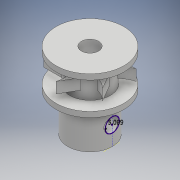
# Autodesk Inventor part: wheelSpindle
Saved by Autodesk Inventor 2018 (Build 220112000, 112)
## iProperties
Created: 2017-10-22
Part Number: wheelSpindle
Material: Generic
Document SubType Name: Modeling
Designer: Prakash
Density: 1 g/cm^3
Appearance: Default
Author: Prakash
Autodesk Inventor part; units mm, degrees
ref_plane "XZ Plane" through (0, 0, 0) normal (0, 1, 0) x (-1, 0, 0)
ref_plane "XY Plane" through (0, 0, 0) normal (0, 0, 1) x (1, 0, 0)
sketch "Sketch1" plane through (0, 0, 0) normal (0, 0, 1) x (1, 0, 0)
  circle A0 centre (0, 0) radius 7.5
  circle A1 centre (0, 0) radius 12.5
  circle A2 centre (0, 0) radius 3.175
  circle A3 centre (0, 0) radius 8.175
  dimension "d18" = 6.35
  dimension "d19" = 16.35
  dimension "d40" = 15
  dimension "d41" = 5
  constraints: 4 centre point, 4 coincident
  measures "d18" diameter of A2
  measures "d19" diameter of A3
  measures "d40" diameter of A0
  measures "d41" radial gap between concentric circles of A1 A0
extrude "Extrusion1" add sketch "Sketch1" along normal blind 14 contours A0 | A2
extrude "Extrusion2" add sketch "Sketch1" along normal blind 2 contours A1 | A3
sketch "Sketch2" plane through (0, 0, 14) normal (0, 0, 1) x (1, 0, 0)
  circle A0 centre (0, 0) radius 7.5 projected
  circle A1 centre (0, 0) radius 12.5 projected
extrude "Extrusion3" add sketch "Sketch2" against normal blind 2
ref_plane "Work Plane1" through (0, 0, 7) normal (0, 0, -1) x (-1, 0, 0)
extrude "Extrusion5" cut sketch "Sketch1" along normal up to surface (14 mm away) contours A2
extrude "Extrusion6" add sketch "Sketch1" against normal blind 14 contours A0 | A3
ref_plane "Work Plane2" through (8.175, 0, 0) normal (1, 0, 0) x (0, 1, 0)
sketch "Sketch9" plane through (0, 0, 7) normal (0, 0, -1) x (-1, 0, 0)
  circle A0 centre (0, 0) radius 7.5 projected
  line L0 (0, -7.5) -> (0, -12.5) construction
  circle A1 centre (0, 0) radius 12.5 projected
  arc A2 (0, -7.5) -> (0, -12.5) centre (7.5993, -10) ccw
  line L1 (0, -12.5) -> (-3.3398, -6.7154)
  circle A3 centre (0, 0) radius 7.5
  line L2 (6.4952, -3.75) -> (10.8253, -6.25) construction
  line L3 (10.8253, -6.25) -> (4.1458, -6.25)
  arc A4 (6.4952, -3.75) -> (10.8253, -6.25) centre (12.4599, 1.5812) ccw
  line L4 (6.4952, 3.75) -> (10.8253, 6.25) construction
  line L5 (10.8253, 6.25) -> (7.4855, 0.4654)
  arc A5 (6.4952, 3.75) -> (10.8253, 6.25) centre (4.8606, 11.5812) ccw
  line L6 (0, 7.5) -> (0, 12.5) construction
  line L7 (0, 12.5) -> (3.3398, 6.7154)
  arc A6 (0, 7.5) -> (0, 12.5) centre (-7.5993, 10) ccw
  line L8 (-6.4952, 3.75) -> (-10.8253, 6.25) construction
  line L9 (-10.8253, 6.25) -> (-4.1458, 6.25)
  arc A7 (-6.4952, 3.75) -> (-10.8253, 6.25) centre (-12.4599, -1.5812) ccw
  line L10 (-6.4952, -3.75) -> (-10.8253, -6.25) construction
  line L11 (-10.8253, -6.25) -> (-7.4855, -0.4654)
  arc A8 (-6.4952, -3.75) -> (-10.8253, -6.25) centre (-4.8606, -11.5812) ccw
  point P0 (0, -10)
  point P1 (8.6603, -5)
  point P2 (8.6603, 5)
  point P3 (0, 10)
  point P4 (-8.6603, 5)
  point P5 (-8.6603, -5)
  dimension "d58" = 8
  dimension "d59" = 30
  dimension "d62" = 360
  constraints: 24 end point, 12 point on circle, 7 centre point, 2 vertical, 1 coincident, 1 midpoint, 1 vertical alignment, 64 other
  measures "d58" radius of A2
  measures "d59" angle of L1 L0
extrude "Extrusion9" add sketch "Sketch9" along normal mid plane 4 contours A0 A5 L5 | A4 L3 A0 | A0 A6 L7 | A2 L1 A0 | L9 A0 A7 | L11 A0 A8
sketch "Sketch10" plane through (8.175, 0, 0) normal (1, 0, 0) x (0, 1, 0)
  line L0 (0, 0) -> (0, -14) construction
  line L1 (3.175, -14) -> (-3.175, -14) construction
  circle A0 centre (0, -7) radius 2.6543
  circle A1 centre (0, -7) radius 2.5273
  dimension "d67" = 5.3086
  dimension "d68" = 5.0546
  constraints: 2 centre point, 2 end point, 2 midpoint, 1 coincident
  measures "d67" diameter of A0
  measures "d68" diameter of A1
extrude "Extrusion10" cut sketch "Sketch10" against normal blind 3.81 contours A1
loft "Loft1" cut profiles "Sketch10" section 2 edges at (4.365, -2.5273, -7) contours A0 | A1
body "Solid1"
